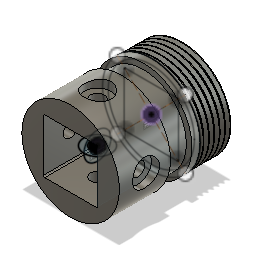
Top_Adapter_FFB (Autodesk Fusion 360 design; units mm, degrees)
Autodesk Fusion 360 part; units mm, degrees
sketch "Sketch1" plane through (0, 0, 0) normal (0, 0, 1) x (1, 0, 0)
  circle A0 centre (0, 0) radius 18.1
  circle A1 centre (0, 0) radius 16
  line L0 (-9.6, 10.1) -> (9.6, 10.1)
  line L1 (10.1, 9.6) -> (10.1, -9.6)
  line L2 (9.6, -10.1) -> (-9.6, -10.1)
  line L3 (-10.1, -9.6) -> (-10.1, 9.6)
  line L4 (-10.1, 10.1) -> (10.1, -10.1) construction
  line L5 (10.1, 10.1) -> (-10.1, -10.1) construction
  line L6 (-12.64, 12.64) -> (12.64, -12.64) construction
  line L7 (12.64, 12.64) -> (-12.64, -12.64) construction
  arc A2 (10.1, 9.6) -> (9.6, 10.1) centre (9.6, 9.6) ccw
  arc A3 (9.6, -10.1) -> (10.1, -9.6) centre (9.6, -9.6) ccw
  arc A4 (-10.1, -9.6) -> (-9.6, -10.1) centre (-9.6, -9.6) ccw
  arc A5 (-9.6, 10.1) -> (-10.1, 9.6) centre (-9.6, 9.6) ccw
  dimension "d1" = 36.2
  dimension "d4" = 32
  dimension "d5" = 20.2
  dimension "d6" = 20.2
  dimension "d7" = 25.28
  dimension "d8" = 25.28
  dimension "d19" = 0.5
  constraint coincident A0.centre A1.centre
  constraint concentric A0 A1
  constraint horizontal L0
  constraint perpendicular L0 L1
  constraint parallel L0 L2
  constraint parallel L1 L3
  constraint coincident L4 A0.centre
  constraint coincident L5 A0.centre
  constraint coincident L6 A0.centre
  constraint coincident L7 A0.centre
  constraint coincident L5.start L0
  constraint coincident L5.start L1
  constraint tangent L0 A2
  constraint tangent L1 A2
  constraint coincident L4.end L2
  constraint coincident L4.end L1
  constraint tangent L2 A3
  constraint tangent L1 A3
  constraint equal A2 A3
  constraint coincident L5.end L2
  constraint coincident L5.end L3
  constraint tangent L2 A4
  constraint tangent L3 A4
  constraint equal A2 A4
  constraint coincident L4.start L0
  constraint coincident L4.start L3
  constraint tangent L0 A5
  constraint tangent L3 A5
  constraint equal A2 A5
  measures "d1" diameter of A0
  measures "d4" diameter of A1
  measures "d5" distance of L4.end L5.end
  measures "d6" distance of L5.start L4.end
  measures "d7" distance of L6.start L7.end
  measures "d8" distance of L6.end L7.end
  measures "d19" radius of A2
extrude "Extrude1" add sketch "Sketch1" against normal blind 12 contours A0 | A1 | L0 L1 L2 L3 A2 A3 A4 A5 makes body 1
thread "Thread1" "ISO Metric profile 36.0 M36x2 6g" major diameter 35.822 minor diameter 33.529 pitch 2 angle 60 modelled right hand crest width 0.2818 on face at (18.0775, -0.9022, -8) crest through (17.911, 0, 0.5) on bodies 1
extrude "Extrude2" add sketch "Sketch1" along normal blind 30 separate body contours A0 | A1 | L0 L1 L2 L3 A2 A3 A4 A5 makes body 2
sketch "Sketch4" plane through (0, 0, 0) normal (1, 0, 0) x (0, 0, -1)
extrude "Extrude4" cut sketch "Sketch1" along normal blind 8 from surface at 3 contours A0 bodies 2
sketch "Sketch5" plane through (0, 0, 0) normal (1, 0, 0) x (0, 0, -1)
  circle A0 centre (-20.0001, 0) radius 2.6
  circle A1 centre (-20.0001, 0) radius 5
  dimension "d24" = 5.2
  dimension "d26" = 10
  dimension "d27" = 20.0001
  constraint concentric A0 A1
  constraint horizontal origin A0.centre
  measures "d24" diameter of A0
  measures "d26" diameter of A1
  measures "d27" distance of A0.centre origin
extrude "Extrude5" cut sketch "Sketch5" along normal through all and the other way through all contours A0 bodies 2
extrude "Extrude6" cut sketch "Sketch5" against normal blind 4 from surface at 19 bodies 2
extrude "Extrude7" cut sketch "Sketch5" along normal blind 4 from surface at -19 bodies 2
sketch "Sketch6" plane through (0, 0, -12) normal (0, 0, -1) x (-1, 0, 0)
  line L0 (0, 0) -> (-8.4018, 0) construction
  line L1 (0, 0) -> (0, -5.9373) construction
  circle A0 centre (0, 0) radius 11.25
  line L2 (10.1, 10.1) -> (-10.1, -10.1) construction
  line L3 (-10.1, 10.1) -> (10.1, -10.1) construction
  arc A1 (-10.1, -9.6) -> (-9.6, -10.1) centre (-9.6, -9.6) ccw
  arc A2 (9.6, -10.1) -> (10.1, -9.6) centre (9.6, -9.6) ccw
  arc A3 (10.1, 9.6) -> (9.6, 10.1) centre (9.6, 9.6) ccw
  arc A4 (-9.6, 10.1) -> (-10.1, 9.6) centre (-9.6, 9.6) ccw
  arc A5 (-10.87, 2.8992) -> (-10.87, -2.8992) centre (-10.8, 0) ccw
  arc A6 (-4.0993, -10.4766) -> (4.0993, -10.4766) centre (0, -10.4) ccw
  arc A7 (10.87, -2.8992) -> (10.87, 2.8992) centre (10.8, 0) ccw
  arc A8 (4.0993, 10.4766) -> (-4.0993, 10.4766) centre (0, 10.4) ccw
  line L4 (-9.6, -10.1) -> (-4.955, -10.1)
  line L5 (4.955, -10.1) -> (9.6, -10.1)
  line L6 (-10.1, 9.6) -> (-10.1, 4.955)
  line L7 (-10.1, -4.955) -> (-10.1, -9.6)
  line L8 (9.6, 10.1) -> (4.955, 10.1)
  line L9 (-4.955, 10.1) -> (-9.6, 10.1)
  line L10 (10.1, -9.6) -> (10.1, -4.955)
  line L11 (10.1, 4.955) -> (10.1, 9.6)
  spline S0 degree 3 poles (7.6713, -16.185) (9.7341, -15.1284) (11.5719, -13.6814) (14.5676, -10.1818) (15.7046, -8.17) (17.13, -3.8481) (17.4145, -1.5832) (17.0963, 2.9004) (16.5071, 5.0765) (14.8558, 8.4071) (14.0257, 9.645) (12.0718, 11.8627) (10.9589, 12.835) (9.7334, 13.6495) knots 0 0 0 0 0.695282 0.695282 1.382357 1.382357 2.061224 2.061224 2.731881 2.731881 3.177609 3.177609 3.619591 3.619591 3.619591 3.619591
  arc A9 (9.7334, 13.6495) -> (-9.7334, 13.6495) centre (0, 0) ccw
  spline S1 degree 3 poles (-9.7334, 13.6495) (-11.5619, 12.4343) (-13.1338, 10.8716) (-15.6103, 7.211) (-16.4822, 5.1426) (-17.395, 0.7612) (-17.4167, -1.5116) (-16.5875, -5.9665) (-15.7342, -8.1036) (-13.6582, -11.3181) (-12.6516, -12.5012) (-10.3483, -14.5849) (-9.0592, -15.4741) (-7.6713, -16.185) knots 0 0 0 0 0.658659 0.658659 1.325519 1.325519 2.000579 2.000579 2.683837 2.683837 3.147341 3.147341 3.614584 3.614584 3.614584 3.614584
  arc A10 (-7.6713, -16.185) -> (7.6713, -16.185) centre (0, 0) ccw
  dimension "d34" = 8.2
  dimension "d35" = 10.4
  dimension "d36" = 5.8
  dimension "d37" = 10.8
  dimension "d38" = 22.5
  dimension "d39" = 20.2
  dimension "d40" = 20.2
  dimension "d41" = 0.5
  constraint coincident L0.start L1.start
  constraint horizontal L0
  constraint perpendicular L0 L1
  constraint symmetric L0 A6 A8
  constraint horizontal L0.start A7.centre
  constraint vertical A8.centre L0.start
  constraint symmetric L1 A5 A7
  constraint horizontal L8
  constraint perpendicular L6 L8
  constraint parallel L4 L8
  constraint parallel L6 L10
  constraint coincident L2 L0.start
  constraint coincident L3 L0.start
  constraint coincident L2.end L6
  constraint coincident L2.end L4
  constraint tangent A1 L6
  constraint tangent A1 L4
  constraint coincident L3.end L4
  constraint coincident L3.end L10
  constraint tangent A2 L4
  constraint tangent A2 L10
  constraint equal A1 A2
  constraint coincident L2.start L10
  constraint coincident L2.start L8
  constraint tangent A3 L10
  constraint tangent A3 L8
  constraint equal A1 A3
  constraint coincident L3.start L8
  constraint coincident L3.start L6
  constraint tangent A4 L8
  constraint tangent A4 L6
  constraint equal A1 A4
  constraint collinear L4 L5
  constraint collinear L6 L7
  constraint collinear L8 L9
  constraint collinear L10 L11
  constraint coincident A0 L11.start
  constraint coincident A0 A7.end
  constraint coincident A0 A7.start
  constraint coincident A0 L10.end
  constraint coincident A0 A6.end
  constraint coincident A0 L5.start
  constraint coincident A0 A6.start
  constraint coincident A0 L4.end
  constraint coincident A0 A5.end
  constraint coincident A0 L7.start
  constraint coincident A0 L6.end
  constraint coincident A0 A5.start
  constraint coincident A0 A8.end
  constraint coincident A0 L9.start
  constraint coincident A0 L8.end
  constraint coincident A0 A8.start
  measures "d34" diameter of A8
  measures "d35" distance of A8.centre L0.start
  measures "d36" diameter of A7
  measures "d37" distance of L1 A7.centre
  measures "d38" diameter of A0
  measures "d39" distance of L2.end L3.end
  measures "d40" distance of L3.start L2.end
  measures "d41" radius of A1
extrude "Extrude8" cut sketch "Sketch6" against normal blind 4 contours A0 | A0 A7 | A0 A8 | A0 A6 | A0 A5 bodies 1
extrude "Extrude9" cut sketch "Sketch1" along normal mid plane 66 contours L0 L1 L2 L3 A2 A3 A4 A5 bodies 1 2
sketch "Sketch7" plane through (10.1, 0, 0) normal (-1, 0, 0) x (0, 0, 1)
  line L0 (30, -9.6) -> (30, 9.6)
  line L1 (30, 9.6) -> (0, 9.6)
  line L2 (0, 9.6) -> (0, -9.6)
  line L3 (0, -9.6) -> (30, -9.6)
  circle A0 centre (20.0001, 0) radius 2.6
sketch "Sketch8" plane through (0, 0, 0) normal (0, 1, 0) x (1, 0, 0)
  circle A0 centre (0, -20.0001) radius 2.6
  circle A1 centre (0, -20.0001) radius 5
  point P0 (0, -20.0001)
  dimension "d46" = 5.2
  dimension "d47" = 10
  constraint coincident P0 A0.centre
  constraint concentric A0 A1
  measures "d46" diameter of A0
  measures "d47" diameter of A1
extrude "Extrude10" cut sketch "Sketch8" along normal through all and the other way through all contours A0 bodies 2
extrude "Extrude11" cut sketch "Sketch8" against normal blind 4 from surface at 19 bodies 2
extrude "Extrude12" cut sketch "Sketch8" along normal blind 4 from surface at -19 bodies 2
equation "d6 = d5"
equation "d7 = d6 + 0.2 in"
equation "d8 = d7"
equation "d34 = ( 4.1 * 2 ) * 1 mm"
equation "d35 = ( 20.8 / 2 ) * 1 mm"
equation "d36 = 2.9 * 2 mm"
equation "d37 = ( 21.6 / 2 ) * 1 mm"
